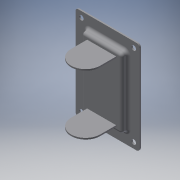
# Autodesk Inventor part: WallMount
Saved by Autodesk Inventor 2018 (Build 220105000, 105)
## iProperties
Created: 2004-11-28
Document SubType Name: Modeling
Designer: Autodesk, Inc.
Manufacturer: Standard
Standards Organization: Custom
Description: SWING ARM WALL MOUNT
Mass: 35.0537 g
Surface Area: 194.518 cm^2
Volume: 35.0537 cm^3
Density: 1 g/cm^3
Material: Generic
Appearance: Default
CAGE: 1LJX3
Dept. ID: Product Design
Description #2: ---
Finish #1: ---
Finish #2: ---
Material ID: ---
Project Number: ---
Author: Autodesk, Inc.
Autodesk Inventor part; units mm, degrees
ref_plane "YZ Plane" through (0, 0, 0) normal (1, 0, 0) x (0, 1, 0)
ref_plane "XZ Plane" through (0, 0, 0) normal (0, 1, 0) x (-1, 0, 0)
sketch "Sketch2" plane through (0, 0, 0) normal (0, 0, 1) x (1, 0, 0)
  line L0 (-31.75, 50.8) -> (31.75, 50.8)
  line L1 (34.925, 47.625) -> (34.925, -47.625)
  line L2 (31.75, -50.8) -> (-31.75, -50.8)
  line L3 (-34.925, -47.625) -> (-34.925, 47.625)
  arc A0 (-31.75, 50.8) -> (-34.925, 47.625) centre (-31.75, 47.625) ccw
  arc A1 (34.925, 47.625) -> (31.75, 50.8) centre (31.75, 47.625) ccw
  arc A2 (31.75, -50.8) -> (34.925, -47.625) centre (31.75, -47.625) ccw
  arc A3 (-34.925, -47.625) -> (-31.75, -50.8) centre (-31.75, -47.625) ccw
  point P0 (0, 0)
  point P1 (-34.925, 50.8)
  point P2 (34.925, -50.8)
  point P3 (34.925, 50.8)
  point P4 (-34.925, -50.8)
  point P5 (-34.925, 0)
  point P6 (0, 50.8)
  dimension "d0" = 69.85
  dimension "d1" = 101.6
  dimension "d4" = 3.175
  constraints: 8 end point, 8 point on circle, 8 point on line, 8 tangent, 4 centre point, 3 equal radius, 2 midpoint, 2 parallel, 1 horizontal, 1 horizontal alignment, 1 perpendicular, 1 vertical alignment
  measures "d0" distance of point (34.925, -50.8) point (-34.925, -50.8)
  measures "d1" distance of point (-34.925, -50.8) point (-34.925, 50.8)
  measures "d4" radius of A0
extrude "Extrusion1" add sketch "Sketch2" along normal blind 1.524
sketch "Sketch3" plane through (0, 0, 1.524) normal (0, 0, 1) x (1, 0, 0)
  line L0 (-19.05, 38.1) -> (19.05, 38.1)
  line L1 (22.225, 34.925) -> (22.225, -34.925)
  line L2 (19.05, -38.1) -> (-19.05, -38.1)
  line L3 (-22.225, -34.925) -> (-22.225, 34.925)
  arc A0 (-19.05, 38.1) -> (-22.225, 34.925) centre (-19.05, 34.925) ccw
  arc A1 (22.225, 34.925) -> (19.05, 38.1) centre (19.05, 34.925) ccw
  arc A2 (19.05, -38.1) -> (22.225, -34.925) centre (19.05, -34.925) ccw
  arc A3 (-22.225, -34.925) -> (-19.05, -38.1) centre (-19.05, -34.925) ccw
  line L4 (31.75, -50.8) -> (-31.75, -50.8) projected
  line L5 (-34.925, -47.625) -> (-34.925, 47.625) projected
  point P0 (0, 0)
  point P1 (0, 38.1)
  point P2 (-22.225, 0)
  dimension "d7" = 3.175
  dimension "d8" = 12.7
  dimension "d9" = 12.7
  constraints: 8 end point, 8 point on circle, 8 tangent, 4 centre point, 3 equal radius, 2 midpoint, 2 parallel, 1 horizontal, 1 horizontal alignment, 1 perpendicular, 1 vertical alignment
  measures "d7" radius of A0
  measures "d8" distance between parallel lines of L4 L2
  measures "d9" distance between parallel lines of L5 L3
extrude "Extrusion2" add sketch "Sketch3" along normal blind 6.35
fillet "Fillet1" radius 3.175 16 edges at (0, 38.1, 7.874) (21.2951, 37.1701, 7.874) (22.225, 0, 7.874) (21.2951, -37.1701, 7.874) (0, -38.1, 7.874) (-21.2951, -37.1701, 7.874) (-22.225, 0, 7.874) (-21.2951, 37.1701, 7.874) (0, 38.1, 1.524) (21.2951, 37.1701, 1.524) (22.225, 0, 1.524) (21.2951, -37.1701, 1.524) (0, -38.1, 1.524) (-21.2951, -37.1701, 1.524) (-22.225, 0, 1.524) (-21.2951, 37.1701, 1.524)
ref_plane "Work Plane1" through (0, -31.75, 0) normal (0, 1, 0) x (-1, 0, 0)
sketch "Sketch4" plane through (0, -31.75, 0) normal (0, 1, 0) x (-1, 0, 0)
  line L0 (-15.875, 0) -> (15.875, 0)
  line L1 (15.875, 0) -> (15.875, 25.4)
  line L2 (15.875, 25.4) -> (-15.875, 25.4)
  line L3 (-15.875, 25.4) -> (-15.875, 0)
  circle A0 centre (0, 25.4) radius 15.875
  line L4 (-31.75, 0) -> (31.75, 0) projected
  point P0 (0, 0)
  point P1 (0, 0)
  point P2 (0, 0)
  dimension "d15" = 31.75
  dimension "d14" = 25.4
  constraints: 8 end point, 3 midpoint, 2 parallel, 1 coincident, 1 collinear, 1 horizontal, 1 horizontal alignment, 1 perpendicular, 2 other
  measures "d14" distance between parallel lines of L2 L0
extrude "Extrusion3" add sketch "Sketch4" against normal blind 1.524
mirror "Mirror1" about plane through (0, 0, 0) normal (0, 1, 0) of "Extrusion3"
sketch "Sketch5" plane through (0, 0, 1.524) normal (0, 0, 1) x (1, 0, 0)
  circle A0 centre (-28.575, -44.45) radius 2.54
  line L0 (-34.925, -47.625) -> (-34.925, 47.625) projected
  line L1 (31.75, -50.8) -> (-31.75, -50.8) projected
  point P0 (0, 0)
  dimension "d18" = 5.08
  dimension "d19" = 6.35
  dimension "d20" = 6.35
  constraints: 1 centre point
  measures "d18" diameter of A0
  measures "d19" distance from line of L0 A0.centre
  measures "d20" distance from line of L1 A0.centre
extrude "Extrusion4" cut sketch "Sketch5" against normal through all
mirror "Mirror2" about plane through (0, 0, 0) normal (0, 1, 0) of "Extrusion4"
mirror "Mirror3" about plane through (0, 0, 0) normal (1, 0, 0) of "Extrusion4", "Mirror2"
body "Solid1"
